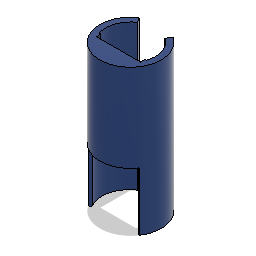
Battery_endspacer_2023.04.01 (Autodesk Fusion 360 design; units mm, degrees)
Autodesk Fusion 360 part; units mm, degrees
sketch "Sketch1" plane through (0, 0, 0) normal (0, 1, 0) x (1, 0, 0)
  circle A0 centre (0, 0) radius 10.5
  circle A1 centre (0, -0.5) radius 9.25
  line L0 (8, 12) -> (0, 0)
  line L1 (0, 0) -> (-8, 12)
  line L2 (-12, -8) -> (0, 0)
  line L3 (0, 0) -> (12, -8)
  circle A2 centre (0, 0) radius 8.5
  line L4 (6, 8) -> (6, -7)
  line L5 (-6, 8) -> (-6, -7)
  point P0 (0, -0.5)
  dimension "d1" = 21
  dimension "d2" = 0.5
  dimension "d3" = 18.5
  dimension "d4" = 17
  constraint coincident A0.centre L0.end
  constraint vertical A0.centre A1.centre
  constraint coincident P0 A1.centre
  constraint vertical L4
  constraint vertical L5
  measures "d1" diameter of A0
  measures "d2" distance of A0.centre P0
  measures "d3" diameter of A1
  measures "d4" diameter of A2
extrude "Extrude1" add sketch "Sketch1" along normal blind 30 contours A0 A1 L0 L3 | A0 A1 L2 L3 | A0 A1 L1 L2 | A1 L0 A2 L4 | A1 L3 A2 L4 | A1 L2 L3 A2 | A1 L1 A2 L5 | A1 L2 A2 L5
extrude "Extrude2" add sketch "Sketch1" against normal blind 20 contours A0 A1 L0 L3 | A0 A1 L1 L2
extrude "Extrude3" add sketch "Sketch1" along normal blind 2 contours L3 A2 L4 | L3 A2 L4 | L2 A2 L5 | L2 A2 L5
chamfer "Chamfer1" distance 1.5 angle 45 1 edges at (8.5, 2, 0)
chamfer "Chamfer1" distance 1.5 angle 45 1 edges at (-8.5, 2, 0)
sketch "Sketch2" plane through (0, 30, 0) normal (0, 1, 0) x (-1, 0, 0)
  arc A0 (5.8244, -8.7365) -> (-5.8244, -8.7365) centre (0, 0) ccw
  line L0 (-5.8244, -8.7365) -> (-4.715, -7.0724)
  arc A1 (4.715, -7.0724) -> (-4.715, -7.0724) centre (0, 0) ccw
  line L1 (4.715, -7.0724) -> (5.8244, -8.7365)
  circle A2 centre (0, 0) radius 10.5
  line L2 (12, 4.2) -> (-14.4146, 4.2)
  line L3 (7.3899, 4.2) -> (-7.3899, 4.2)
  line L4 (5.9974, 4.2) -> (5.9974, 6.0234)
  line L5 (-6.0026, 4.2) -> (-6.0026, 6.0182)
  line L6 (7.5, 2.7) -> (-7.5, 2.7)
  line L7 (-7.5, 2.7) -> (-7.5, 4.2)
  line L8 (-7.5, 4.2) -> (7.5, 4.2)
  line L9 (7.5, 4.2) -> (7.5, 2.7)
  line L10 (11.5236, 2.7) -> (-11.5285, 2.7)
  point P0 (7.3899, 4.2)
  point P1 (0, 4.2)
  dimension "d13" = 21
  dimension "d16" = 4.2
  dimension "d27" = 15
  dimension "d28" = 1.5
  constraint horizontal L2
  constraint coincident A1 P0
  constraint coincident L2 P0
  constraint horizontal L3
  constraint coincident P0 L3.start
  constraint coincident L3 L4.start
  constraint coincident A1 L4.end
  constraint perpendicular L2 L4
  constraint coincident L3 L5.start
  constraint coincident A1 L5.end
  constraint perpendicular L3 L5
  constraint horizontal L6
  constraint vertical L7
  constraint horizontal L8
  constraint vertical L9
  constraint midpoint L8 P1
  constraint coincident L3 P1
  constraint vertical A0.centre P1
  constraint horizontal L10
  measures "d13" diameter of A2
  measures "d16" vertical distance of A0.centre L2.end
  measures "d27" distance of L6.start L6.end
  measures "d28" distance of L6.start L8.end
extrude "Extrude4" add sketch "Sketch2" against normal blind 8 contours A1 L2 L3 L4 L8 | A1 L2 L3 L4 L5 L8 | A1 L2 L3 L5 L8
extrude "Extrude5" add sketch "Sketch2" against normal blind 30 contours A1 L9 L10 | A1 L7 L10 | A1 L2 L3 L4 L8 | A1 L2 L3 L5 L8
extrude "Extrude6" cut sketch "Sketch2" against normal blind 30 contours A1 L2 L8 L9 | A1 L2 L7 L8
